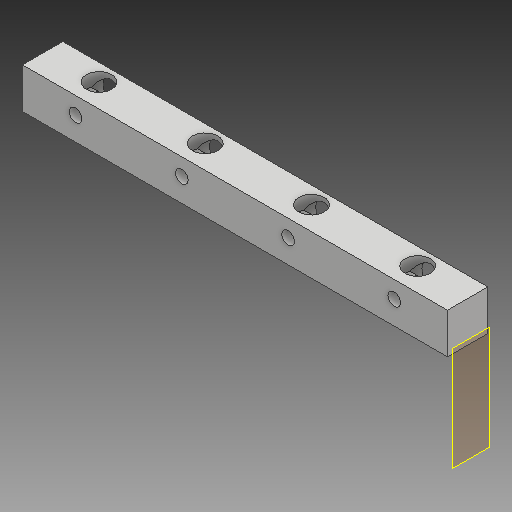
# Autodesk Inventor part: 30_Connector_Baseplate
Saved by Autodesk Inventor 2019 (Build 230136000, 136)
## iProperties
Created: 2018-07-12
Part Number: 30_Connector_Baseplate
Material: Generisch
Document SubType Name: Modeling
Designer: diederichbenedict
Density: 1 g/cm^3
Appearance: Vorgabe
Author: diederichbenedict
Autodesk Inventor part; units mm, degrees
ref_plane "YZ Plane" through (0, 0, 0) normal (1, 0, 0) x (0, 1, 0)
ref_plane "XZ Plane" through (0, 0, 0) normal (0, 1, 0) x (-1, 0, 0)
ref_plane "XY Plane" through (0, 0, 0) normal (0, 0, 1) x (1, 0, 0)
ref_plane "Arbeitsebene1" through (50, 0, 0) normal (1, 0, 0) x (0, 0, -1)
sketch "Skizze1" plane through (50, 0, 0) normal (1, 0, 0) x (0, 0, -1)
  line L0 (100, 0) -> (100, 8) projected
  line L1 (-9.5, -101.5) -> (-1.5, -101.5) projected
  line L2 (0, -1.5) -> (-9.5, -1.5)
  line L3 (-9.5, -1.5) -> (-9.5, 8)
  line L4 (-9.5, 8) -> (0, 8)
  line L5 (0, 8) -> (0, -1.5)
  point P0 (0, 0)
  constraints: 8 end point, 2 parallel, 1 horizontal, 1 perpendicular, 1 other
extrude "Extrusion1" add sketch "Skizze1" against normal blind 50
sketch "Skizze2" plane through (50, -1.5, 9.5) normal (0, 0, 1) x (1, 0, 0)
  circle A0 centre (-12.5, 5.5) radius 1.75 projected
  circle A1 centre (-37.5, 5.5) radius 1.75 projected
  point P0 (-50, 1.5)
hole "Bohrung1" at (37.5, 4, 9.5) at (12.5, 4, 9.5) direction (0, 0, -1) diameter 3 end through all counterbore diameter 6 counterbore depth 3
sketch "Skizze3" plane through (50, 8, 9.5) normal (0, 1, 0) x (1, 0, 0)
  circle A0 centre (-12.5, 4) radius 1.75 projected
  circle A1 centre (-37.5, 4) radius 1.75 projected
  point P0 (-50, 9.5)
hole "Bohrung2" at (37.5, 8, 5.5) at (12.5, 8, 5.5) direction (0, -1, 0) diameter 3 end through all counterbore diameter 6 counterbore depth 3
mirror "Spiegeln1" about plane through (0, 3.25, 4.75) normal (-1, 0, 0) of "Bohrung1", "Extrusion1", "Bohrung2"
